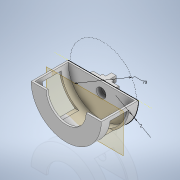
# Autodesk Inventor part: Winddingshalter
Saved by Autodesk Inventor 2022 (Build 260153000, 153)
## iProperties
Created: 2024-04-17
Part Number: Winddingshalter
Material: Generic
Document SubType Name: Modeling
Designer: Gotham City
Density: 1 g/cm^3
Appearance: Default
Author: Gotham City
Autodesk Inventor part; units mm, degrees
ref_plane "YZ Plane" through (0, 0, 0) normal (1, 0, 0) x (0, 1, 0)
ref_plane "XZ Plane" through (0, 0, 0) normal (0, 1, 0) x (-1, 0, 0)
ref_plane "XY Plane" through (0, 0, 0) normal (0, 0, 1) x (1, 0, 0)
sketch "Sketch1" plane through (0, 0, 0) normal (0, 0, 1) x (1, 0, 0)
  arc A0 (-37, 0) -> (37, 0) centre (0, 0) ccw
  line L0 (-51.8, 0) -> (51.8, 0) construction
  circle A1 centre (0, 0) radius 35 construction
  line L1 (-37, 0) -> (37, 0)
  dimension "d1" = 70
  dimension "d2" = 2
  constraints: 2 centre point, 2 coincident, 2 end point, 2 point on circle, 2 point on line, 1 collinear
  measures "d1" diameter of A1
  measures "d2" radial gap between concentric circles of A0 A1
extrude "Extrusion1" add sketch "Sketch1" along normal blind 2
sketch "Sketch2" plane through (0, 0, 2) normal (0, 0, 1) x (1, 0, 0)
  arc A0 (-37, 0) -> (37, 0) centre (0, 0) ccw projected
  arc A1 (-35, 0) -> (35, 0) centre (0, 0) ccw
  line L0 (37, 0) -> (-37, 0) projected
  line L1 (-37, 0) -> (37, 0)
  dimension "d5" = 2
  constraints: 2 end point, 2 point on circle, 1 centre point, 1 horizontal
  measures "d5" radial gap between concentric circles of A0 A1
extrude "Extrusion2" add sketch "Sketch2" along normal blind 35 contours L0 A1 A0
ref_plane "Work Plane1" through (0, 0, 19.5) normal (0, 0, 1) x (1, 0, 0)
mirror "Mirror1" about plane through (0, 0, 19.5) normal (0, 0, 1) of "Extrusion1"
sketch "Sketch3" plane through (0, 0, 39) normal (0, 0, 1) x (1, 0, 0)
  circle A0 centre (0, 0) radius 21
  dimension "d8" = 42
  constraints: 1 centre point, 1 coincident
  measures "d8" diameter of A0
extrude "Extrusion3" cut sketch "Sketch3" against normal blind 35
sketch "Sketch4" plane through (0, 0, 0) normal (1, 0, 0) x (0, 1, 0)
  line L0 (-4, 9.5) -> (-31, 9.5)
  line L1 (-31, 9.5) -> (-31, 29.5)
  line L2 (-31, 29.5) -> (-4, 29.5)
  line L3 (-4, 29.5) -> (-4, 9.5)
  line L4 (-44.4, 19.5) -> (7.4, 19.5) construction
  line L5 (0, 0) -> (0, 39) construction
  line L6 (-35, 37) -> (-35, 2) construction
  dimension "d11" = 20
  dimension "d12" = 4
  dimension "d13" = 4
  constraints: 8 end point, 2 parallel, 1 horizontal, 1 perpendicular, 1 other
  measures "d11" distance of L2.end L0.start
  measures "d12" distance between parallel lines of L5 L3
  measures "d13" distance between parallel lines of L1 L6
extrude "Extrusion4" cut sketch "Sketch4" along normal through all both and the other way through all
sketch "Sketch5" plane through (0, 0, 0) normal (0, 1, 0) x (-1, 0, 0)
  line L0 (37, 0) -> (-37, 0) projected
  line L1 (0, -31.0583) -> (0, 50.6764) construction
  line L2 (-6, -3) -> (6, -3)
  line L3 (6, -3) -> (6, -5.2)
  line L4 (6, -5.2) -> (-6, -5.2)
  line L5 (-6, -5.2) -> (-6, -3)
  line L6 (-2.5, -5.2) -> (2.5, -5.2)
  line L7 (2.5, -5.2) -> (2.5, -11.2)
  line L8 (2.5, -11.2) -> (-2.5, -11.2)
  line L9 (-2.5, -11.2) -> (-2.5, -5.2)
  line L10 (0, -3) -> (0, -11.2) construction
  line L11 (-37, 0) -> (37, 0) construction
  line L12 (-13.75, 0) -> (13.75, 0)
  line L13 (13.75, 0) -> (13.75, -3)
  line L14 (13.75, -3) -> (-13.75, -3)
  line L15 (-13.75, -3) -> (-13.75, 0)
  dimension "d32" = 2.2
  dimension "d33" = 3.5
  dimension "d34" = 6
  dimension "d35" = 5
  dimension "d36" = 27.5
  dimension "d37" = 3
  constraints: 26 end point, 6 parallel, 3 horizontal, 3 midpoint, 3 perpendicular, 3 point on line, 1 vertical, 1 other
  measures "d32" distance of L4.end L2.start
  measures "d33" distance between parallel lines of L9 L5
  measures "d34" distance of L8.end L6.start
  measures "d35" distance of L7.end L8.end
  measures "d36" distance of L13.end L14.end
  measures "d37" distance of L14.end L12.start
extrude "Extrusion5" add sketch "Sketch5" against normal blind 30
sketch "Sketch6" plane through (0, 0, 2) normal (0, 0, 1) x (1, 0, 0)
  line L0 (0, 0) -> (0, -21) construction
  arc A0 (-21, 0) -> (21, 0) centre (0, 0) ccw projected
  point P0 (0, -10.5)
  constraints: 2 end point, 1 midpoint, 1 point on circle, 1 vertical
hole "Hole1" at (0, -10.5, 2) direction (0, 0, -1) diameter 5.5 end through all counterbore diameter 10 counterbore depth 5 clearance for "Socket Head Cap Screw ISO 4762" size "M5" standard "ISO"
sketch "Sketch7" plane through (-2.5, -30, -11.2) normal (-1, 0, 0) x (0, 0, 1)
  line L0 (6, 30) -> (6, 0) projected
  line L1 (0, 30) -> (0, 20.6456) projected
  line L2 (0, 18.3544) -> (0, 0) projected
  line L3 (0, 15) -> (6, 15)
  line L4 (6, 15) -> (6, 24)
  line L5 (6, 24) -> (0, 24)
  line L6 (0, 24) -> (0, 15)
  line L7 (6, 18.3544) -> (0, 18.3544) construction
  line L8 (0, 19.5) -> (6, 19.5) construction
  line L9 (6, 15) -> (0, 9)
  line L10 (0, 15) -> (0, 9)
  line L11 (0, 20.6456) -> (6, 20.6456) construction
  point P0 (11.2, 30)
  point P1 (0, 24)
  dimension "d39" = 9
  dimension "d41" = 1.1456
  dimension "d42" = 45
  dimension "d45" = 1.1456
  constraints: 14 end point, 3 point on line, 2 midpoint, 2 parallel, 2 perpendicular, 1 collinear, 1 horizontal, 1 other
  measures "d39" distance between parallel lines of L5 L3
  measures "d41" distance between parallel lines of L8 L7
  measures "d42" angle of L0 L9
  measures "d45" distance between parallel lines of L11 L8
extrude "Extrusion6" cut sketch "Sketch7" along normal through all both and the other way through all
equation "\"d13\" = d12"
equation "\"d45\" = d41"
body "Solid1"
